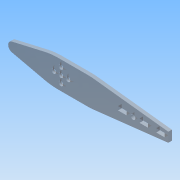
# Autodesk Inventor part: leg
Saved by Autodesk Inventor 2015 (Build 190159000, 159)
## iProperties
Created: 2016-01-28
Part Number: leg
Material: Plastique PMMA
Document SubType Name: Tôlerie
Designer: Gregwar
Density: 1.188 g/cm^3
Sheet Metal Rule: Par défaut_mm
Appearance: Polycarbonate - Transparent
Author: Gregwar
Autodesk Inventor part; units mm, degrees
ref_plane "YZ Plane" through (0, 0, 0) normal (1, 0, 0) x (0, 1, 0)
ref_plane "XZ Plane" through (0, 0, 0) normal (0, 1, 0) x (-1, 0, 0)
ref_plane "XY Plane" through (0, 0, 0) normal (0, 0, 1) x (1, 0, 0)
sketch "Esquisse1" plane through (0, 0, 0) normal (0, 1, 0) x (-1, 0, 0)
  line L0 (8, 11.5) -> (-90, 11.5)
  line L1 (-90, 11.5) -> (-90, -11.5)
  line L2 (-90, -11.5) -> (8, -11.5)
  line L3 (8, -11.5) -> (8, 11.5)
  line L4 (0, 11.5) -> (0, -11.5) construction
  line L5 (8, 11.5) -> (45, 3)
  line L6 (45, 3) -> (45, -3)
  line L7 (45, -3) -> (8, -11.5)
  point P0 (0, 0)
  point P1 (0, 0)
  dimension "d0" = 23
  dimension "d1" = 8
  dimension "d3" = 90
  dimension "d4" = 45
  dimension "d5" = 6
  measures "d0" distance between parallel lines of L0 L2
  measures "d1" distance between parallel lines of L4 L3
  measures "d3" distance from line of L1 point (0, 0)
  measures "d4" distance from line of point (0, 0) L6
  measures "d5" distance of L5.end L6.end
extrude "Plaque1" add sketch "Esquisse1" along normal blind 3
sketch "Esquisse2" plane through (0, 3, 0) normal (0, 1, 0) x (1, 0, 0)
  line L0 (0, 0) -> (-6, 0) construction
  point P0 (0, -6)
  point P1 (6, 0)
  point P2 (0, 6)
  dimension "d9" = 360
  dimension "d11" = 6
  constraints: 2 end point, 1 coincident, 1 horizontal, 5 other
  measures "d11" distance of point (0, 0) L0.end
hole "Perçage1" at (0, 3, 0) at (-6, 3, 0) at (0, 3, 6) at (6, 3, 0) at (0, 3, -6) direction (0, -1, 0) diameter 3.8 end through all counterbore diameter 5.5 counterbore depth 1
sketch "Esquisse3" plane through (0, 3, 0) normal (0, 1, 0) x (1, 0, 0)
  circle A0 centre (6, 0) radius 2.75 construction
  circle A1 centre (-6, 0) radius 2.75 construction
  circle A2 centre (0, 0) radius 2.75 construction
  circle A3 centre (0, -6) radius 2.75 construction
  circle A4 centre (0, 6) radius 2.75 construction
  line L0 (-8, -11.5) -> (-45, -3) construction
  line L1 (90, -11.5) -> (-8, -11.5) construction
  line L2 (90, 11.5) -> (90, -11.5) construction
  line L3 (-8, 11.5) -> (90, 11.5) construction
  line L4 (-45, 3) -> (-8, 11.5) construction
  line L5 (-45, -3) -> (-45, 3) construction
  line L6 (90, -11.5) -> (90, 11.5) projected
  line L7 (90, -4) -> (25, -11.5)
  line L8 (90, -11.5) -> (90, -4)
  line L9 (90, -11.5) -> (25, -11.5)
  line L10 (-8, -11.5) -> (90, -11.5) projected
  line L11 (90, 0) -> (18.7328, 0) construction
  line L12 (90, 4) -> (25, 11.5)
  line L13 (90, 11.5) -> (90, 4)
  line L14 (90, 11.5) -> (25, 11.5)
  dimension "d19" = 8
  dimension "d20" = 65
  constraints: 14 end point, 2 collinear, 2 point on line, 2 symmetric about line, 1 horizontal, 1 midpoint
  measures "d19" distance of L12.start L7.start
  measures "d20" distance from line of L13 L12.end
extrude "Couper1" cut sketch "Esquisse3" against normal through all
fillet "Congé1" radius 50 4 edges at (25, 1.5, 11.5) (-8, 1.5, 11.5) (25, 1.5, -11.5) (-8, 1.5, -11.5)
fillet "Congé2" radius 4 2 edges at (-45, 1.5, -3) (-45, 1.5, 3)
sketch "Esquisse4" plane through (0, 3, 0) normal (0, 1, 0) x (1, 0, 0)
  arc A0 (-41.0891, 3.8985) -> (-41.0891, -3.8985) centre (-40.1935, 0) ccw construction
  line L0 (-13.5255, -10.2306) -> (-41.0891, -3.8985) construction
  arc A1 (-13.5255, -10.2306) -> (-2.3306, -11.5) centre (-2.3306, 38.5) ccw construction
  line L1 (22.1249, -11.5) -> (-2.3306, -11.5) construction
  arc A2 (22.1249, -11.5) -> (27.8561, -11.1704) centre (22.1249, 38.5) ccw construction
  line L2 (27.8561, -11.1704) -> (90, -4) construction
  line L3 (90, 4) -> (90, -4) construction
  line L4 (90, 4) -> (27.8561, 11.1704) construction
  arc A3 (27.8561, 11.1704) -> (22.1249, 11.5) centre (22.1249, -38.5) ccw construction
  line L5 (-2.3306, 11.5) -> (22.1249, 11.5) construction
  arc A4 (-2.3306, 11.5) -> (-13.5255, 10.2306) centre (-2.3306, -38.5) ccw construction
  line L6 (-41.0891, 3.8985) -> (-13.5255, 10.2306) construction
  circle A5 centre (0, 6) radius 2.75 construction
  circle A6 centre (0, -6) radius 2.75 construction
  circle A7 centre (0, 0) radius 2.75 construction
  circle A8 centre (-6, 0) radius 2.75 construction
  circle A9 centre (6, 0) radius 2.75 construction
  line L7 (90, -4) -> (90, 4) construction
  line L8 (90, 4) -> (90, -4) construction
  line L9 (90, 0) -> (71.2936, 0) construction
  line L10 (79.9, 1.575) -> (87, 1.575)
  line L11 (87, 1.575) -> (87, -1.575)
  line L12 (87, -1.575) -> (79.9, -1.575)
  line L13 (79.9, -1.575) -> (79.9, 1.575)
  line L14 (79.9, 0) -> (87, 0) construction
  line L15 (76, 0) -> (57.2936, 0) construction
  line L16 (65.9, 1.575) -> (73, 1.575)
  line L17 (73, 1.575) -> (73, -1.575)
  line L18 (73, -1.575) -> (65.9, -1.575)
  line L19 (65.9, -1.575) -> (65.9, 1.575)
  line L20 (65.9, 0) -> (73, 0) construction
  line L21 (72, 0) -> (53.2936, 0) construction
  line L22 (47.9, -1.575) -> (47.9, 1.575)
  line L23 (55, 1.575) -> (55, -1.575)
  line L24 (55, -1.575) -> (47.9, -1.575)
  line L25 (47.9, 0) -> (55, 0) construction
  line L26 (58, 0) -> (39.2936, 0) construction
  line L27 (47.9, 1.575) -> (55, 1.575)
  line L28 (55, 0) -> (65.9, 0) construction
  circle A10 centre (60.45, 0) radius 2.05
  point P0 (61.8782, 0)
  dimension "d46" = 3.15
  dimension "d47" = 3
  dimension "d48" = 7.1
  dimension "d51" = 14
  dimension "d58" = 18
  dimension "d63" = 4.1
  constraints: 40 end point, 4 horizontal, 4 midpoint, 3 collinear, 2 parallel, 2 perpendicular, 1 centre point, 29 other
  measures "d46" distance of L10.end L11.end
  measures "d47" distance between parallel lines of L3 L11
  measures "d48" distance of L10.start L10.end
  measures "d51" distance of L10.start L19.end
  measures "d58" distance of L19.end L22.end
  measures "d63" diameter of A10
extrude "Couper2" cut sketch "Esquisse4" against normal blind 3
equation "\"d12\" = ollo_hole"
equation "\"d14\" = ollo_ring"
equation "\"d15\" = ollo_depth"
equation "\"d17\" = Epaisseur"
equation "\"d21\" = Epaisseur"
equation "\"d44\" = Epaisseur"
equation "\"LargeurGrugeage\" = Epaisseur"
equation "\"ProfondeurGrugeage\" = 0.5 * Epaisseur"
equation "\"TailleGrugeage\" = 4 * Epaisseur"
equation "\"RestesMinimum\" = 2 * Epaisseur"
equation "\"Rayondetransition\" = RayonPli"
equation "\"TailleRayonJacobi\" = RayonPli"
equation "\"TailleJeu\" = Epaisseur"
equation "\"d6\" = RayonPli"
equation "\"ollo_hole\" = 3.8"
equation "\"ollo_ring\" = 5.5"
equation "\"ollo_depth\" = 1"
equation "\"Epaisseur\" = 3"
equation "\"RayonPli\" = 4"
